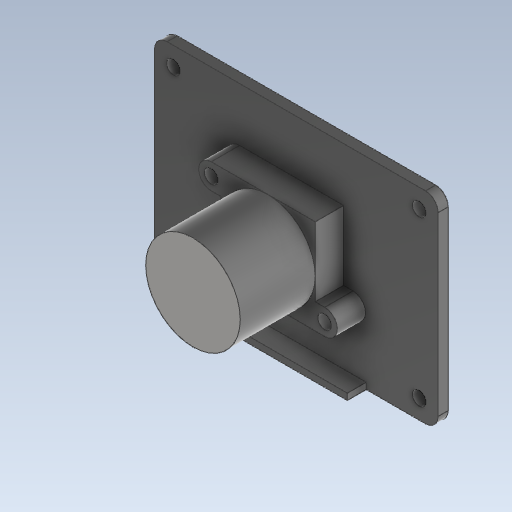
# Autodesk Inventor part: KBCR-S02MU
Saved by Autodesk Inventor 2020.4 (Build 244396000, 396)
## iProperties
Part Number: KBCR-S02MU
Material: 一般
Document SubType Name: Modeling
Designer: Masato Kubotera
Density: 2.20183 g/cm^3
Appearance: 滑らか - 黒
Mass: 10.8 g
Surface Area: 34.0637 cm^2
Volume: 4.90502 cm^3
Catalog Web Link: https://www.shikino.co.jp/products/product-kbcr-s02mu.php
Description: ReadyMade
Author: Masato Kubotera
Autodesk Inventor part; units mm, degrees
ref_plane "YZ Plane" through (0, 0, 0) normal (1, 0, 0) x (0, 1, 0)
ref_plane "XZ Plane" through (0, 0, 0) normal (0, 1, 0) x (-1, 0, 0)
ref_plane "XY Plane" through (0, 0, 0) normal (0, 0, 1) x (1, 0, 0)
sketch "スケッチ1" plane through (0, 0, 0) normal (0, 0, 1) x (1, 0, 0)
  line L0 (14, 22.5) -> (-14, 22.5)
  line L1 (-16, 20.5) -> (-16, -20.5)
  line L2 (-14, -22.5) -> (14, -22.5)
  line L3 (16, -20.5) -> (16, 20.5)
  line L4 (16, 22.5) -> (-16, -22.5) construction
  line L5 (-16, 22.5) -> (16, -22.5) construction
  line L6 (-13, 19.5) -> (13, 19.5) construction
  line L7 (13, 19.5) -> (13, -19.5) construction
  line L8 (13, -19.5) -> (-13, -19.5) construction
  line L9 (-13, -19.5) -> (-13, 19.5) construction
  line L10 (-13, 19.5) -> (13, -19.5) construction
  line L11 (13, 19.5) -> (-13, -19.5) construction
  circle A0 centre (-13, -19.5) radius 1.1
  line L12 (-16, 0) -> (16, 0) construction
  line L13 (0, 22.5) -> (0, -22.5) construction
  circle A1 centre (-13, 19.5) radius 1.1
  circle A2 centre (13, -19.5) radius 1.1
  circle A3 centre (13, 19.5) radius 1.1
  circle A4 centre (-13, -19.5) radius 2 construction
  circle A5 centre (-13, 19.5) radius 2 construction
  circle A6 centre (13, -19.5) radius 2 construction
  circle A7 centre (13, 19.5) radius 2 construction
  circle A8 centre (0, 0) radius 7.5
  circle A9 centre (-5.5, -9) radius 1.1
  circle A10 centre (-5.5, -9) radius 2
  line L14 (-7.5, -9) -> (-7.5, 7.5)
  line L15 (-7.5, 7.5) -> (3.5, 7.5)
  line L16 (-3.5, -9) -> (-3.5, -7.5)
  circle A11 centre (5.5, 9) radius 2
  line L17 (3.5, 9) -> (3.5, 7.5)
  circle A12 centre (5.5, 9) radius 1.1
  line L18 (7.5, 9) -> (7.5, -7.5)
  line L19 (7.5, -7.5) -> (-3.5, -7.5)
  arc A13 (-16, -20.5) -> (-14, -22.5) centre (-14, -20.5) ccw
  arc A14 (14, -22.5) -> (16, -20.5) centre (14, -20.5) ccw
  arc A15 (16, 20.5) -> (14, 22.5) centre (14, 20.5) ccw
  arc A16 (-14, 22.5) -> (-16, 20.5) centre (-14, 20.5) ccw
  line L20 (16, -11.1) -> (15, -11.1)
  line L21 (15, -11.1) -> (15, 11.1)
  line L22 (16, 11.1) -> (15, 11.1)
  point P0 (-3.5, -7.5)
  point P1 (0, -7.5)
  point P2 (-7.5, 0)
  point P3 (7.5, 0)
  point P4 (0, 7.5)
  point P5 (3.5, 7.5)
  dimension "d0" = 32
  dimension "d1" = 45
  dimension "d5" = 2.2
  dimension "d6" = 4
  dimension "d11" = 2.2
  dimension "d12" = 4
  dimension "d20" = 360
  dimension "d22" = 11
  dimension "d34" = 2
  dimension "d37" = 22.2
  dimension "d38" = 1
  dimension "d39" = 18
  dimension "d40" = 26
  dimension "d41" = 39
  constraints: 46 end point, 17 centre point, 12 point on circle, 12 tangent, 9 point on line, 8 midpoint, 8 symmetric about line, 6 coincident, 4 horizontal, 4 parallel, 3 equal radius, 3 perpendicular, 2 vertical, 31 other
  measures "d0" distance of L5.end L4.end
  measures "d1" distance of L4.end L5.start
  measures "d5" diameter of A0
  measures "d6" diameter of A4
  measures "d11" diameter of A9
  measures "d12" diameter of A10
  measures "d22" horizontal distance of A11.centre A9.centre
  measures "d34" radius of A13
  measures "d37" distance of L22.start L20.start
  measures "d38" distance of L20.start L20.end
  measures "d39" vertical distance of A11.centre A10.centre
  measures "d40" distance of L7.end L8.end
  measures "d41" distance of L8.end L6.start
extrude "押し出し1" add sketch "スケッチ1" along normal blind 1.6 contours A15 L3 L22 L21 L20 A14 L2 A13 L1 A16 L0 | L3 L20 L21 L22 | A8 | L18 L19 A8 | A8 L15 L17 A11 L18 | A8 L14 L15 | L19 L16 A10 L14 A8 | A11 | A10
extrude "押し出し2" add sketch "スケッチ1" along normal blind 4.6 contours L3 L20 L21 L22
extrude "押し出し3" add sketch "スケッチ1" along normal blind 6.1 contours L18 L19 A8 | A8 L15 L17 A11 L18 | A8 L14 L15 | L19 L16 A10 L14 A8 | A11 | A10
extrude "押し出し4" add sketch "スケッチ1" along normal blind 18 contours A8
extrude "押し出し5" add sketch "スケッチ1" against normal blind 2 contours A11 | A10 | A9 | A12
